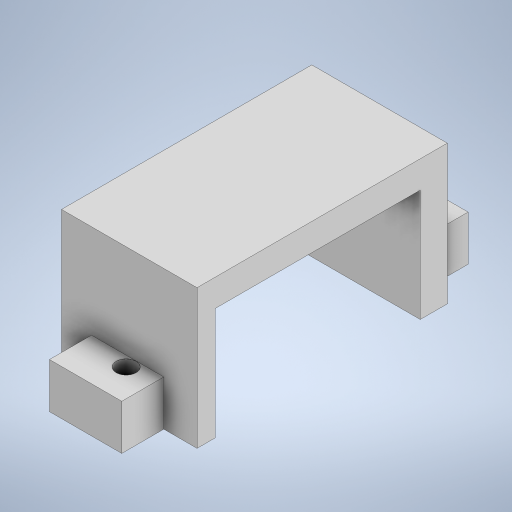
# Autodesk Inventor part: Sostiene motor
Saved by Autodesk Inventor 2024 (Build 280153000, 153)
## iProperties
Created: 2024-04-28
Part Number: Sostiene motor
Material: Generic
Document SubType Name: Modeling
Designer: samue
Density: 1 g/cm^3
Appearance: Default
Author: samue
## iProperties of the stored document Sostiene motor_3DPrint.ipt
Created: 2024-04-28
Part Number: Sostiene motor_3DPrint
Material: Generic
Document SubType Name: Modeling
Designer: samue
Density: 1 g/cm^3
Appearance: Default
Author: samue
Autodesk Inventor part; units mm, degrees
ref_plane "YZ Plane" through (0, 0, 0) normal (1, 0, 0) x (0, 1, 0)
ref_plane "XZ Plane" through (0, 0, 0) normal (0, 1, 0) x (-1, 0, 0)
ref_plane "XY Plane" through (0, 0, 0) normal (0, 0, 1) x (1, 0, 0)
sketch "Sketch1" plane through (0, 0, 0) normal (0, 1, 0) x (-1, 0, 0)
  line L0 (7.5, 11.35) -> (-7.5, 11.35)
  line L1 (-7.5, 11.35) -> (-7.5, -11.35)
  line L2 (-7.5, -11.35) -> (7.5, -11.35)
  line L3 (7.5, -11.35) -> (7.5, 11.35)
  line L4 (7.5, 11.35) -> (-7.5, -11.35) construction
  line L5 (-7.5, 11.35) -> (7.5, -11.35) construction
  point P0 (0, 0)
  dimension "d0" = 15
  dimension "d1" = 22.7
  constraints: 12 end point, 2 midpoint, 2 parallel, 1 horizontal, 1 perpendicular
  measures "d0" distance of L2.end L1.end
  measures "d1" distance of L1.end L0.end
extrude "Extrusion1" add sketch "Sketch1" along normal blind 3
sketch "Sketch2" plane through (0, 3, 0) normal (0, 1, 0) x (1, 0, 0)
  line L0 (-7.5, 11.35) -> (-7.5, -11.35) projected
  line L1 (-7.5, -11.35) -> (7.5, -11.35)
  line L2 (7.5, -11.35) -> (7.5, -13.35)
  line L3 (7.5, -13.35) -> (-7.5, -13.35)
  line L4 (-7.5, -13.35) -> (-7.5, -11.35)
  line L5 (-7.5, 11.35) -> (7.5, 11.35)
  line L6 (7.5, 11.35) -> (7.5, 14.35)
  line L7 (7.5, 14.35) -> (-7.5, 14.35)
  line L8 (-7.5, 14.35) -> (-7.5, 11.35)
  point P0 (0, 0)
  dimension "d4" = 15
  dimension "d5" = 2
  dimension "d6" = 3
  constraints: 16 end point, 4 parallel, 2 horizontal, 2 perpendicular, 1 point on line
  measures "d4" distance of L2.end L3.end
  measures "d5" distance of L1.end L2.end
  measures "d6" distance of L6.end L5.end
extrude "Extrusion2" add sketch "Sketch2" against normal blind 15.4
sketch "Sketch3" plane through (-7.5, 3, 13.35) normal (0, 0, 1) x (1, 0, 0)
  line L0 (3.3204, -10.4) -> (11.3204, -10.4)
  line L1 (11.3204, -10.4) -> (11.3204, -15.4)
  line L2 (3.3204, -15.4) -> (3.3204, -10.4)
  line L3 (15, -15.4) -> (0, -15.4) projected
  line L4 (3.3204, -10.4) -> (7.5, -15.4) construction
  line L5 (11.3204, -10.4) -> (7.5, -15.4) construction
  line L6 (3.3204, -15.4) -> (11.3204, -15.4)
  point P0 (7.5, -3)
  dimension "d9" = 8
  dimension "d10" = 5
  constraints: 12 end point, 3 point on line, 1 horizontal, 1 midpoint, 1 parallel, 1 perpendicular
  measures "d9" distance of L0.start L0.end
  measures "d10" distance between parallel lines of L0 L3
extrude "Extrusion3" add sketch "Sketch3" along normal blind 4.65
sketch "Sketch4" plane through (-4.1796, -7.4, 13.35) normal (0, 1, 0) x (1, 0, 0)
  circle A0 centre (4.9615, -1.1239) radius 1.1
  point P0 (4.1796, 13.35)
  dimension "d13" = 2.2
  constraints: 1 centre point
  measures "d13" diameter of A0
extrude "Extrusion4" cut sketch "Sketch4" against normal blind 6.4
sketch "Sketch5" plane through (7.5, 3, -14.35) normal (0, 0, -1) x (-1, 0, 0)
  line L0 (10.6996, -10.4559) -> (2.6996, -10.4559)
  line L1 (2.6996, -10.4559) -> (2.6996, -15.4559)
  line L2 (10.6996, -15.4559) -> (10.6996, -10.4559)
  line L3 (7.8181, -10.4) -> (7.8181, -15.4) projected
  line L4 (10.6996, -10.4559) -> (7.8181, -15.4559) construction
  line L5 (2.6996, -10.4559) -> (7.8181, -15.4559) construction
  line L6 (10.6996, -15.4559) -> (2.6996, -15.4559)
  point P0 (7.5, -3)
  point P1 (6.6996, -15.4559)
  point P2 (6.6996, -10.4559)
  dimension "d16" = 8
  dimension "d18" = 5
  constraints: 12 end point, 2 midpoint, 2 point on line, 1 horizontal, 1 parallel, 1 perpendicular
  measures "d16" distance of L0.start L0.end
  measures "d18" distance of point (6.7, -15.456) point (6.7, -10.456)
extrude "Extrusion5" add sketch "Sketch5" along normal blind 5
sketch "Sketch6" plane through (-3.1996, -7.4559, -14.35) normal (0, 1, 0) x (1, 0, 0)
  circle A0 centre (3.9961, 1.8138) radius 1.1
  point P0 (3.1996, -14.35)
  dimension "d21" = 2.2
  constraints: 1 centre point
  measures "d21" diameter of A0
extrude "Extrusion6" cut sketch "Sketch6" against normal blind 5
body "Solid1"
